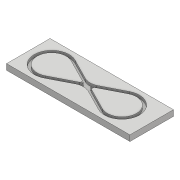
# Autodesk Inventor part: Part5
Saved by Autodesk Inventor 2017 (Build 210142000, 142)
## iProperties
Created: 2019-07-04
Part Number: Part5
Material: Generic
Document SubType Name: Modeling
Designer: Admin
Density: 1 g/cm^3
Appearance: Default
Author: Admin
Autodesk Inventor part; units mm, degrees
ref_plane "YZ Plane" through (0, 0, 0) normal (1, 0, 0) x (0, 1, 0)
ref_plane "XZ Plane" through (0, 0, 0) normal (0, 1, 0) x (-1, 0, 0)
ref_plane "XY Plane" through (0, 0, 0) normal (0, 0, 1) x (1, 0, 0)
sketch "Sketch1" plane through (0, 0, 0) normal (0, 0, 1) x (1, 0, 0)
  arc A0 (-237.2727, 94.5362) -> (-237.2727, 5.4638) centre (-260, 50) ccw
  line L0 (-160.4727, 44.6557) -> (-237.2727, 5.4638)
  line L1 (-160.4727, 55.3443) -> (-237.2727, 94.5362)
  arc A1 (-232.7273, 103.4434) -> (-232.7273, -3.4434) centre (-260, 50) ccw
  line L2 (-232.7273, -3.4434) -> (-157.7465, 34.8201)
  line L3 (-157.7465, 65.1799) -> (-232.7273, 103.4434)
  line L4 (84.5, -25) -> (-340.5, -25)
  line L5 (-340.5, -25) -> (-340.5, 125)
  line L6 (-340.5, 125) -> (84.5, 125)
  line L7 (84.5, 125) -> (84.5, -25)
  line L8 (84.5, -25) -> (-340.5, 125) construction
  line L9 (-340.5, -25) -> (84.5, 125) construction
  arc A2 (-40.7273, 5.4638) -> (-40.7273, 94.5362) centre (-18, 50) ccw
  line L10 (-118.2834, 45.0415) -> (-40.7273, 5.4638)
  arc A3 (-45.2727, -3.4434) -> (-45.2727, 103.4434) centre (-18, 50) ccw
  line L11 (-45.2727, -3.4434) -> (-120.2535, 34.8201)
  line L12 (-120.2535, 65.1799) -> (-45.2727, 103.4434)
  arc A4 (-157.7465, 65.1799) -> (-120.2535, 65.1799) centre (-139, 111.5326) ccw
  arc A5 (-120.2535, 34.8201) -> (-157.7465, 34.8201) centre (-139, -11.5326) ccw
  arc A6 (-160.4727, 44.6557) -> (-160.4727, 55.3443) centre (-163.2, 50) ccw
  circle A7 centre (-153.117, 50) radius 2
  arc A8 (-153.117, 53.699) -> (-153.117, 46.3109) centre (-153.0877, 50.0049) ccw
  line L13 (-153.117, 53.699) -> (-149.5823, 52.9955)
  line L14 (-149.5823, 52.9955) -> (-139, 38.4674)
  line L15 (-139, 38.4674) -> (-143.9506, 38.3782)
  line L16 (-143.9506, 38.3782) -> (-153.117, 46.3109)
  circle A9 centre (-124.4918, 50) radius 2
  arc A10 (-124.4918, 46.3109) -> (-124.4918, 53.699) centre (-124.5211, 50.0049) ccw
  line L17 (-124.4918, 53.699) -> (-128.0265, 52.9955)
  line L18 (-128.0265, 52.9955) -> (-138.6089, 38.4674)
  line L19 (-138.6089, 38.4674) -> (-133.6583, 38.3782)
  line L20 (-133.6583, 38.3782) -> (-124.4918, 46.3109)
  arc A11 (-118.3602, 54.9193) -> (-118.2834, 45.0415) centre (-107.4722, 50.0647) ccw
  line L21 (-118.3602, 54.9193) -> (-40.7273, 94.5362)
  point P0 (0, 0)
  dimension "d3" = 10
  dimension "d4" = 425
  dimension "d5" = 150
  dimension "d6" = 50
  dimension "d7" = 6
  dimension "d8" = 4
  constraints: 44 end point, 21 point on circle, 12 centre point, 4 tangent, 2 parallel, 1 horizontal, 1 perpendicular
  measures "d3" distance between parallel lines of L1 L3
  measures "d4" distance of L5.end L6.end
  measures "d5" distance of L4.end L5.end
  measures "d6" radius of A4
  measures "d7" radius of A6
  measures "d8" diameter of A7
extrude "Extrusion1" add sketch "Sketch1" along normal blind 10 contours L1 A6 L0 A0 | L4 L5 L6 L7 | L10 A11 L21 A2
extrude "Extrusion2" add sketch "Sketch1" along normal blind 10 separate body contours L18 L17 A10 L20 L19
extrude "Extrusion3" add sketch "Sketch1" along normal blind 10 separate body contours L15 L16 A8 L13 L14 A5 | A5 L15
sketch "Sketch2" plane through (0, 0, 0) normal (0, 0, -1) x (-1, 0, 0)
  line L0 (340.5, 125) -> (-84.5, 125) projected
  line L1 (340.5, -25) -> (340.5, 125) projected
  line L2 (-84.5, 125) -> (340.5, 125)
  line L3 (340.5, 125) -> (340.5, -25)
  line L4 (340.5, -25) -> (-84.5, -25)
  line L5 (-84.5, -25) -> (-84.5, 125)
  point P0 (0, 0)
  constraints: 8 end point, 2 parallel, 1 horizontal, 1 perpendicular
extrude "Extrusion4" add sketch "Sketch2" along normal blind 10 bodies 1
fillet "Fillet1" radius 6.25 2 edges at (-118.3602, 54.9193, 5) (-118.2834, 45.0415, 5)
extrude "Extrusion5" add sketch "Sketch1" along normal blind 9 separate body contours A7
extrude "Extrusion6" add sketch "Sketch1" along normal blind 9 separate body contours A9
combine bodies "Combine1" operation type add bodies to combine 5 1
combine bodies "Combine2" operation type add bodies to combine 4 5
body "Solid2"
body "Solid3"
body "Solid4"
